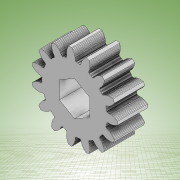
# Autodesk Inventor part: Piñon
Saved by Autodesk Inventor 2022 (Build 260153000, 153)
## iProperties
Created: 2022-03-01
Part Number: Piñon
Material: Genérico
Document SubType Name: Modeling
Designer: Marco
Density: 1 g/cm^3
Appearance: Valor por defecto
Author: Marco
Autodesk Inventor part; units mm, degrees
(part 1 of 2)
ref_plane "YZ Plane" through (0, 0, 0) normal (1, 0, 0) x (0, 1, 0)
ref_plane "XZ Plane" through (0, 0, 0) normal (0, 1, 0) x (-1, 0, 0)
ref_plane "XY Plane" through (0, 0, 0) normal (0, 0, 1) x (1, 0, 0)
sketch "Boceto1" plane through (0, 0, 0) normal (0, 0, 1) x (1, 0, 0)
  line L0 (7.7981, 3.0207) -> (7.6871, 2.8757)
  line L1 (7.6871, 2.8757) -> (7.5784, 2.7454)
  line L2 (7.5784, 2.7454) -> (7.4724, 2.6287)
  line L3 (7.4724, 2.6287) -> (7.3713, 2.5262)
  line L4 (7.3713, 2.5262) -> (7.2722, 2.434)
  line L5 (7.2722, 2.434) -> (7.181, 2.3559)
  line L6 (7.181, 2.3559) -> (7.096, 2.2892)
  line L7 (7.096, 2.2892) -> (7.0182, 2.2331)
  line L8 (7.0182, 2.2331) -> (6.9491, 2.1876)
  line L9 (6.9491, 2.1876) -> (6.8365, 2.1229)
  line L10 (6.8365, 2.1229) -> (6.7437, 2.0808)
  line L11 (6.7437, 2.0808) -> (6.6884, 2.066)
  line L12 (6.6884, 2.066) -> (6.5779, 2.0306)
  line L13 (6.5779, 2.0306) -> (6.4822, 1.9901)
  line L14 (6.4822, 1.9901) -> (6.4013, 1.9458)
  line L15 (6.4013, 1.9458) -> (6.3356, 1.8987)
  line L16 (6.3356, 1.8987) -> (6.285, 1.8501)
  line L17 (6.285, 1.8501) -> (6.2496, 1.8011)
  line L18 (6.2496, 1.8011) -> (6.2375, 1.7768)
  line L19 (6.2375, 1.7768) -> (6.2291, 1.7529)
  line L20 (6.2291, 1.7529) -> (6.2245, 1.7295)
  line L21 (6.2245, 1.7295) -> (6.2236, 1.7067)
  line L22 (6.2236, 1.7067) -> (6.2276, 1.6794)
  line L23 (6.2276, 1.6794) -> (6.2912, 1.423)
  line L24 (6.2912, 1.423) -> (6.3092, 1.3409)
  line L25 (6.3092, 1.3409) -> (6.3262, 1.2585)
  line L26 (6.3262, 1.2585) -> (6.3724, 0.9985)
  line L27 (6.3724, 0.9985) -> (6.3799, 0.9719)
  line L28 (6.3799, 0.9719) -> (6.39, 0.9515)
  line L29 (6.39, 0.9515) -> (6.4037, 0.932)
  line L30 (6.4037, 0.932) -> (6.421, 0.9135)
  line L31 (6.421, 0.9135) -> (6.4419, 0.8963)
  line L32 (6.4419, 0.8963) -> (6.4943, 0.8659)
  line L33 (6.4943, 0.8659) -> (6.5603, 0.8421)
  line L34 (6.5603, 0.8421) -> (6.6395, 0.8258)
  line L35 (6.6395, 0.8258) -> (6.7313, 0.8182)
  line L36 (6.7313, 0.8182) -> (6.8353, 0.8202)
  line L37 (6.8353, 0.8202) -> (6.9506, 0.8328)
  line L38 (6.9506, 0.8328) -> (7.0072, 0.8418)
  line L39 (7.0072, 0.8418) -> (7.1091, 0.8411)
  line L40 (7.1091, 0.8411) -> (7.2382, 0.8277)
  line L41 (7.2382, 0.8277) -> (7.3199, 0.8143)
  line L42 (7.3199, 0.8143) -> (7.4138, 0.7947)
  line L43 (7.4138, 0.7947) -> (7.5185, 0.7683)
  line L44 (7.5185, 0.7683) -> (7.6336, 0.7341)
  line L45 (7.6336, 0.7341) -> (7.7617, 0.6901)
  line L46 (7.7617, 0.6901) -> (7.8957, 0.6377)
  line L47 (7.8957, 0.6377) -> (8.04, 0.5742)
  line L48 (8.04, 0.5742) -> (8.1924, 0.4994)
  line L49 (8.1924, 0.4994) -> (8.3528, 0.4121)
  line L50 (8.3528, 0.4121) -> (8.4937, 0.328)
  arc A0 (8.4937, -0.328) -> (8.4937, 0.328) centre (0, 0) ccw
  line L51 (8.4937, -0.328) -> (8.3525, -0.4122)
  line L52 (8.3525, -0.4122) -> (8.1921, -0.4995)
  line L53 (8.1921, -0.4995) -> (8.0398, -0.5743)
  line L54 (8.0398, -0.5743) -> (7.8955, -0.6378)
  line L55 (7.8955, -0.6378) -> (7.7614, -0.6903)
  line L56 (7.7614, -0.6903) -> (7.6334, -0.7343)
  line L57 (7.6334, -0.7343) -> (7.5183, -0.7685)
  line L58 (7.5183, -0.7685) -> (7.4135, -0.7949)
  line L59 (7.4135, -0.7949) -> (7.3197, -0.8145)
  line L60 (7.3197, -0.8145) -> (7.238, -0.828)
  line L61 (7.238, -0.828) -> (7.1089, -0.8413)
  line L62 (7.1089, -0.8413) -> (7.007, -0.842)
  line L63 (7.007, -0.842) -> (6.9504, -0.8331)
  line L64 (6.9504, -0.8331) -> (6.835, -0.8204)
  line L65 (6.835, -0.8204) -> (6.7311, -0.8184)
  line L66 (6.7311, -0.8184) -> (6.6393, -0.8261)
  line L67 (6.6393, -0.8261) -> (6.5601, -0.8424)
  line L68 (6.5601, -0.8424) -> (6.4941, -0.8662)
  line L69 (6.4941, -0.8662) -> (6.4418, -0.8965)
  line L70 (6.4418, -0.8965) -> (6.4209, -0.9138)
  line L71 (6.4209, -0.9138) -> (6.4035, -0.9322)
  line L72 (6.4035, -0.9322) -> (6.3898, -0.9517)
  line L73 (6.3898, -0.9517) -> (6.3797, -0.9722)
  line L74 (6.3797, -0.9722) -> (6.3722, -0.9988)
  line L75 (6.3722, -0.9988) -> (6.326, -1.2588)
  line L76 (6.326, -1.2588) -> (6.309, -1.3412)
  line L77 (6.309, -1.3412) -> (6.291, -1.4233)
  line L78 (6.291, -1.4233) -> (6.2274, -1.6797)
  line L79 (6.2274, -1.6797) -> (6.2234, -1.707)
  line L80 (6.2234, -1.707) -> (6.2243, -1.7298)
  line L81 (6.2243, -1.7298) -> (6.2289, -1.7532)
  line L82 (6.2289, -1.7532) -> (6.2373, -1.7771)
  line L83 (6.2373, -1.7771) -> (6.2493, -1.8014)
  line L84 (6.2493, -1.8014) -> (6.2848, -1.8503)
  line L85 (6.2848, -1.8503) -> (6.3354, -1.899)
  line L86 (6.3354, -1.899) -> (6.4012, -1.946)
  line L87 (6.4012, -1.946) -> (6.482, -1.9904)
  line L88 (6.482, -1.9904) -> (6.5777, -2.0308)
  line L89 (6.5777, -2.0308) -> (6.6882, -2.0662)
  line L90 (6.6882, -2.0662) -> (6.7436, -2.081)
  line L91 (6.7436, -2.081) -> (6.8364, -2.1231)
  line L92 (6.8364, -2.1231) -> (6.9489, -2.1878)
  line L93 (6.9489, -2.1878) -> (7.0181, -2.2333)
  line L94 (7.0181, -2.2333) -> (7.0959, -2.2894)
  line L95 (7.0959, -2.2894) -> (7.1808, -2.3561)
  line L96 (7.1808, -2.3561) -> (7.2721, -2.4341)
  line L97 (7.2721, -2.4341) -> (7.3712, -2.5264)
  line L98 (7.3712, -2.5264) -> (7.4724, -2.6288)
  line L99 (7.4724, -2.6288) -> (7.5784, -2.7455)
  line L100 (7.5784, -2.7455) -> (7.6871, -2.8758)
  line L101 (7.6871, -2.8758) -> (7.7981, -3.0208)
  line L102 (7.7981, -3.0208) -> (7.8928, -3.155)
  arc A1 (7.626, -3.7543) -> (7.8928, -3.155) centre (0, 0) ccw
  line L103 (7.626, -3.7543) -> (7.4628, -3.7736)
  line L104 (7.4628, -3.7736) -> (7.2808, -3.7881)
  line L105 (7.2808, -3.7881) -> (7.1112, -3.7945)
  line L106 (7.1112, -3.7945) -> (6.9535, -3.7939)
  line L107 (6.9535, -3.7939) -> (6.8097, -3.7873)
  line L108 (6.8097, -3.7873) -> (6.6748, -3.7754)
  line L109 (6.6748, -3.7754) -> (6.5557, -3.7598)
  line L110 (6.5557, -3.7598) -> (6.4493, -3.7414)
  line L111 (6.4493, -3.7414) -> (6.3556, -3.721)
  line L112 (6.3556, -3.721) -> (6.2755, -3.7001)
  line L113 (6.2755, -3.7001) -> (6.1521, -3.6598)
  line L114 (6.1521, -3.6598) -> (6.0587, -3.619)
  line L115 (6.0587, -3.619) -> (6.0106, -3.5878)
  line L116 (6.0106, -3.5878) -> (5.9104, -3.5294)
  line L117 (5.9104, -3.5294) -> (5.8163, -3.4853)
  line L118 (5.8163, -3.4853) -> (5.7293, -3.455)
  line L119 (5.7293, -3.455) -> (5.6503, -3.4376)
  line L120 (5.6503, -3.4376) -> (5.5803, -3.4326)
  line L121 (5.5803, -3.4326) -> (5.5202, -3.439)
  line L122 (5.5202, -3.439) -> (5.4941, -3.4462)
  line L123 (5.4941, -3.4462) -> (5.4707, -3.456)
  line L124 (5.4707, -3.456) -> (5.4502, -3.4683)
  line L125 (5.4502, -3.4683) -> (5.4327, -3.4828)
  line L126 (5.4327, -3.4828) -> (5.4151, -3.5041)
  line L127 (5.4151, -3.5041) -> (5.2671, -3.7229)
  line L128 (5.2671, -3.7229) -> (5.2181, -3.7912)
  line L129 (5.2181, -3.7912) -> (5.1682, -3.8589)
  line L130 (5.1682, -3.8589) -> (5.0059, -4.0673)
  line L131 (5.0059, -4.0673) -> (4.9911, -4.0907)
  line L132 (4.9911, -4.0907) -> (4.9827, -4.1119)
  line L133 (4.9827, -4.1119) -> (4.9774, -4.1351)
  line L134 (4.9774, -4.1351) -> (4.9753, -4.1603)
  line L135 (4.9753, -4.1603) -> (4.9765, -4.1874)
  line L136 (4.9765, -4.1874) -> (4.989, -4.2466)
  line L137 (4.989, -4.2466) -> (5.0154, -4.3116)
  line L138 (5.0154, -4.3116) -> (5.0563, -4.3813)
  line L139 (5.0563, -4.3813) -> (5.1121, -4.4547)
  line L140 (5.1121, -4.4547) -> (5.1831, -4.5306)
  line L141 (5.1831, -4.5306) -> (5.2697, -4.6079)
  line L142 (5.2697, -4.6079) -> (5.3142, -4.6439)
  line L143 (5.3142, -4.6439) -> (5.3819, -4.7201)
  line L144 (5.3819, -4.7201) -> (5.4584, -4.825)
  line L145 (5.4584, -4.825) -> (5.503, -4.8947)
  line L146 (5.503, -4.8947) -> (5.5513, -4.9776)
  line L147 (5.5513, -4.9776) -> (5.6018, -5.0731)
  line L148 (5.6018, -5.0731) -> (5.6534, -5.1815)
  line L149 (5.6534, -5.1815) -> (5.7064, -5.3061)
  line L150 (5.7064, -5.3061) -> (5.7571, -5.4408)
  line L151 (5.7571, -5.4408) -> (5.8065, -5.5905)
  line L152 (5.8065, -5.5905) -> (5.8528, -5.7538)
  line L153 (5.8528, -5.7538) -> (5.8953, -5.9314)
  line L154 (5.8953, -5.9314) -> (5.9271, -6.0925)
  arc A2 (5.4396, -6.5315) -> (5.9271, -6.0925) centre (0, 0) ccw
  line L155 (5.4396, -6.5315) -> (5.2825, -6.4827)
  line L156 (5.2825, -6.4827) -> (5.1103, -6.422)
  line L157 (5.1103, -6.422) -> (4.9528, -6.3588)
  line L158 (4.9528, -6.3588) -> (4.809, -6.2941)
  line L159 (4.809, -6.2941) -> (4.6803, -6.2296)
  line L160 (4.6803, -6.2296) -> (4.562, -6.1639)
  line L161 (4.562, -6.1639) -> (4.4595, -6.1012)
  line L162 (4.4595, -6.1012) -> (4.3698, -6.041)
  line L163 (4.3698, -6.041) -> (4.2925, -5.9843)
  line L164 (4.2925, -5.9843) -> (4.2278, -5.9326)
  line L165 (4.2278, -5.9326) -> (4.1315, -5.8456)
  line L166 (4.1315, -5.8456) -> (4.0628, -5.7704)
  line L167 (4.0628, -5.7704) -> (4.0316, -5.7223)
  line L168 (4.0316, -5.7223) -> (3.9638, -5.6282)
  line L169 (3.9638, -5.6282) -> (3.8957, -5.5496)
  line L170 (3.8957, -5.5496) -> (3.8286, -5.4865)
  line L171 (3.8286, -5.4865) -> (3.7635, -5.4385)
  line L172 (3.7635, -5.4385) -> (3.7016, -5.4054)
  line L173 (3.7016, -5.4054) -> (3.644, -5.3869)
  line L174 (3.644, -5.3869) -> (3.6172, -5.3829)
  line L175 (3.6172, -5.3829) -> (3.5919, -5.3823)
  line L176 (3.5919, -5.3823) -> (3.5682, -5.3852)
  line L177 (3.5682, -5.3852) -> (3.5463, -5.3913)
  line L178 (3.5463, -5.3913) -> (3.5215, -5.4036)
  line L179 (3.5215, -5.4036) -> (3.2974, -5.5433)
  line L180 (3.2974, -5.5433) -> (3.2248, -5.5858)
  line L181 (3.2248, -5.5858) -> (3.1517, -5.6274)
  line L182 (3.1517, -5.6274) -> (2.9187, -5.7518)
  line L183 (2.9187, -5.7518) -> (2.8957, -5.7671)
  line L184 (2.8957, -5.7671) -> (2.8794, -5.783)
  line L185 (2.8794, -5.783) -> (2.8651, -5.8021)
  line L186 (2.8651, -5.8021) -> (2.8529, -5.8243)
  line L187 (2.8529, -5.8243) -> (2.843, -5.8495)
  line L188 (2.843, -5.8495) -> (2.8303, -5.9087)
  line L189 (2.8303, -5.9087) -> (2.8281, -5.9788)
  line L190 (2.8281, -5.9788) -> (2.8371, -6.0592)
  line L191 (2.8371, -6.0592) -> (2.8582, -6.1489)
  line L192 (2.8582, -6.1489) -> (2.8922, -6.2471)
  line L193 (2.8922, -6.2471) -> (2.9398, -6.3529)
  line L194 (2.9398, -6.3529) -> (2.9659, -6.4039)
  line L195 (2.9659, -6.4039) -> (2.9967, -6.501)
  line L196 (2.9967, -6.501) -> (3.0239, -6.628)
  line L197 (3.0239, -6.628) -> (3.0364, -6.7098)
  line L198 (3.0364, -6.7098) -> (3.0468, -6.8051)
  line L199 (3.0468, -6.8051) -> (3.0541, -6.9129)
  line L200 (3.0541, -6.9129) -> (3.0571, -7.033)
  line L201 (3.0571, -7.033) -> (3.0548, -7.1683)
  line L202 (3.0548, -7.1683) -> (3.0464, -7.3121)
  line L203 (3.0464, -7.3121) -> (3.0306, -7.4689)
  line L204 (3.0306, -7.4689) -> (3.0065, -7.6369)
  line L205 (3.0065, -7.6369) -> (2.9731, -7.8164)
  line L206 (2.9731, -7.8164) -> (2.9366, -7.9766)
  arc A3 (2.3128, -8.1793) -> (2.9366, -7.9766) centre (0, 0) ccw
  line L207 (2.3128, -8.1793) -> (2.1908, -8.0711)
  line L208 (2.1908, -8.0711) -> (2.0582, -7.9456)
  line L209 (2.0582, -7.9456) -> (1.94, -7.8238)
  line L210 (1.94, -7.8238) -> (1.835, -7.7062)
  line L211 (1.835, -7.7062) -> (1.7437, -7.5949)
  line L212 (1.7437, -7.5949) -> (1.6623, -7.4867)
  line L213 (1.6623, -7.4867) -> (1.5942, -7.3878)
  line L214 (1.5942, -7.3878) -> (1.5367, -7.2963)
  line L215 (1.5367, -7.2963) -> (1.4891, -7.2131)
  line L216 (1.4891, -7.2131) -> (1.4511, -7.1396)
  line L217 (1.4511, -7.1396) -> (1.3985, -7.0209)
  line L218 (1.3985, -7.0209) -> (1.3663, -6.9242)
  line L219 (1.3663, -6.9242) -> (1.3573, -6.8676)
  line L220 (1.3573, -6.8676) -> (1.3337, -6.754)
  line L221 (1.3337, -6.754) -> (1.3034, -6.6546)
  line L222 (1.3034, -6.6546) -> (1.2678, -6.5696)
  line L223 (1.2678, -6.5696) -> (1.2278, -6.4993)
  line L224 (1.2278, -6.4993) -> (1.1847, -6.4439)
  line L225 (1.1847, -6.4439) -> (1.1397, -6.4035)
  line L226 (1.1397, -6.4035) -> (1.1169, -6.389)
  line L227 (1.1169, -6.389) -> (1.094, -6.3782)
  line L228 (1.094, -6.3782) -> (1.0712, -6.3711)
  line L229 (1.0712, -6.3711) -> (1.0486, -6.3678)
  line L230 (1.0486, -6.3678) -> (1.021, -6.369)
  line L231 (1.021, -6.369) -> (0.7594, -6.4054)
  line L232 (0.7594, -6.4054) -> (0.6758, -6.4147)
  line L233 (0.6758, -6.4147) -> (0.5922, -6.423)
  line L234 (0.5922, -6.423) -> (0.3287, -6.4418)
  line L235 (0.3287, -6.4418) -> (0.3014, -6.4464)
  line L236 (0.3014, -6.4464) -> (0.2801, -6.4543)
  line L237 (0.2801, -6.4543) -> (0.2592, -6.4659)
  line L238 (0.2592, -6.4659) -> (0.2391, -6.4813)
  line L239 (0.2391, -6.4813) -> (0.2197, -6.5002)
  line L240 (0.2197, -6.5002) -> (0.1841, -6.5491)
  line L241 (0.1841, -6.5491) -> (0.1535, -6.6123)
  line L242 (0.1535, -6.6123) -> (0.1291, -6.6893)
  line L243 (0.1291, -6.6893) -> (0.1119, -6.7799)
  line L244 (0.1119, -6.7799) -> (0.103, -6.8834)
  line L245 (0.103, -6.8834) -> (0.1034, -6.9994)
  line L246 (0.1034, -6.9994) -> (0.1065, -7.0567)
  line L247 (0.1065, -7.0567) -> (0.0951, -7.1579)
  line L248 (0.0951, -7.1579) -> (0.0683, -7.285)
  line L249 (0.0683, -7.285) -> (0.0464, -7.3648)
  line L250 (0.0464, -7.3648) -> (0.0172, -7.4561)
  line L251 (0.0172, -7.4561) -> (-0.02, -7.5575)
  line L252 (-0.02, -7.5575) -> (-0.0661, -7.6685)
  line L253 (-0.0661, -7.6685) -> (-0.1232, -7.7912)
  line L254 (-0.1232, -7.7912) -> (-0.1894, -7.919)
  line L255 (-0.1894, -7.919) -> (-0.2676, -8.0559)
  line L256 (-0.2676, -8.0559) -> (-0.3579, -8.1996)
  line L257 (-0.3579, -8.1996) -> (-0.4615, -8.35)
  line L258 (-0.4615, -8.35) -> (-0.5599, -8.4815)
  arc A4 (-1.2139, -8.4129) -> (-0.5599, -8.4815) centre (0, 0) ccw
  line L259 (-1.2139, -8.4129) -> (-1.283, -8.2636)
  line L260 (-1.283, -8.2636) -> (-1.353, -8.0949)
  line L261 (-1.353, -8.0949) -> (-1.4115, -7.9356)
  line L262 (-1.4115, -7.9356) -> (-1.4595, -7.7855)
  line L263 (-1.4595, -7.7855) -> (-1.4977, -7.6466)
  line L264 (-1.4977, -7.6466) -> (-1.528, -7.5147)
  line L265 (-1.528, -7.5147) -> (-1.55, -7.3966)
  line L266 (-1.55, -7.3966) -> (-1.5653, -7.2897)
  line L267 (-1.5653, -7.2897) -> (-1.5749, -7.1943)
  line L268 (-1.5749, -7.1943) -> (-1.5798, -7.1116)
  line L269 (-1.5798, -7.1116) -> (-1.5796, -6.9818)
  line L270 (-1.5796, -6.9818) -> (-1.5697, -6.8804)
  line L271 (-1.5697, -6.8804) -> (-1.5548, -6.8251)
  line L272 (-1.5548, -6.8251) -> (-1.5302, -6.7117)
  line L273 (-1.5302, -6.7117) -> (-1.5174, -6.6086)
  line L274 (-1.5174, -6.6086) -> (-1.5154, -6.5164)
  line L275 (-1.5154, -6.5164) -> (-1.5234, -6.4359)
  line L276 (-1.5234, -6.4359) -> (-1.5402, -6.3678)
  line L277 (-1.5402, -6.3678) -> (-1.5649, -6.3126)
  line L278 (-1.5649, -6.3126) -> (-1.5798, -6.29)
  line L279 (-1.5798, -6.29) -> (-1.5964, -6.2708)
  line L280 (-1.5964, -6.2708) -> (-1.6143, -6.2551)
  line L281 (-1.6143, -6.2551) -> (-1.6336, -6.2429)
  line L282 (-1.6336, -6.2429) -> (-1.6593, -6.2328)
  line L283 (-1.6593, -6.2328) -> (-1.9131, -6.1596)
  line L284 (-1.9131, -6.1596) -> (-1.9932, -6.1342)
  line L285 (-1.9932, -6.1342) -> (-2.073, -6.1077)
  line L286 (-2.073, -6.1077) -> (-2.3214, -6.0177)
  line L287 (-2.3214, -6.0177) -> (-2.3482, -6.0109)
  line L288 (-2.3482, -6.0109) -> (-2.3709, -6.0094)
  line L289 (-2.3709, -6.0094) -> (-2.3947, -6.0116)
  line L290 (-2.3947, -6.0116) -> (-2.4193, -6.0174)
  line L291 (-2.4193, -6.0174) -> (-2.4447, -6.0269)
  line L292 (-2.4447, -6.0269) -> (-2.4971, -6.057)
  line L293 (-2.4971, -6.057) -> (-2.5507, -6.1023)
  line L294 (-2.5507, -6.1023) -> (-2.6044, -6.1627)
  line L295 (-2.6044, -6.1627) -> (-2.657, -6.2385)
  line L296 (-2.657, -6.2385) -> (-2.7072, -6.3295)
  line L297 (-2.7072, -6.3295) -> (-2.7539, -6.4356)
  line L298 (-2.7539, -6.4356) -> (-2.7745, -6.4891)
  line L299 (-2.7745, -6.4891) -> (-2.826, -6.577)
  line L300 (-2.826, -6.577) -> (-2.9021, -6.6822)
  line L301 (-2.9021, -6.6822) -> (-2.9546, -6.7462)
  line L302 (-2.9546, -6.7462) -> (-3.0185, -6.8178)
  line L303 (-3.0185, -6.8178) -> (-3.0937, -6.8953)
  line L304 (-3.0937, -6.8953) -> (-3.1809, -6.9779)
  line L305 (-3.1809, -6.9779) -> (-3.283, -7.0668)
  line L306 (-3.283, -7.0668) -> (-3.3955, -7.1566)
  line L307 (-3.3955, -7.1566) -> (-3.5226, -7.2499)
  line L308 (-3.5226, -7.2499) -> (-3.6636, -7.3444)
  line L309 (-3.6636, -7.3444) -> (-3.8194, -7.4396)
  line L310 (-3.8194, -7.4396) -> (-3.9628, -7.5197)
  arc A5 (-4.5309, -7.1917) -> (-3.9628, -7.5197) centre (0, 0) ccw
  line L311 (-4.5309, -7.1917) -> (-4.5332, -7.0275)
  line L312 (-4.5332, -7.0275) -> (-4.5286, -6.8449)
  line L313 (-4.5286, -6.8449) -> (-4.5172, -6.6756)
  line L314 (-4.5172, -6.6756) -> (-4.5001, -6.5189)
  line L315 (-4.5001, -6.5189) -> (-4.4785, -6.3766)
  line L316 (-4.4785, -6.3766) -> (-4.4526, -6.2437)
  line L317 (-4.4526, -6.2437) -> (-4.4246, -6.1269)
  line L318 (-4.4246, -6.1269) -> (-4.3951, -6.023)
  line L319 (-4.3951, -6.023) -> (-4.3651, -5.9319)
  line L320 (-4.3651, -5.9319) -> (-4.3359, -5.8544)
  line L321 (-4.3359, -5.8544) -> (-4.2829, -5.7359)
  line L322 (-4.2829, -5.7359) -> (-4.2326, -5.6473)
  line L323 (-4.2326, -5.6473) -> (-4.1965, -5.6028)
  line L324 (-4.1965, -5.6028) -> (-4.1279, -5.5092)
  line L325 (-4.1279, -5.5092) -> (-4.0742, -5.4202)
  line L326 (-4.0742, -5.4202) -> (-4.035, -5.3369)
  line L327 (-4.035, -5.3369) -> (-4.0094, -5.2601)
  line L328 (-4.0094, -5.2601) -> (-3.9971, -5.1911)
  line L329 (-3.9971, -5.1911) -> (-3.9966, -5.1312)
  line L330 (-3.9966, -5.1312) -> (-4.001, -5.1045)
  line L331 (-4.001, -5.1045) -> (-4.0083, -5.0803)
  line L332 (-4.0083, -5.0803) -> (-4.0184, -5.0586)
  line L333 (-4.0184, -5.0586) -> (-4.031, -5.0396)
  line L334 (-4.031, -5.0396) -> (-4.0503, -5.0199)
  line L335 (-4.0503, -5.0199) -> (-4.2524, -4.8498)
  line L336 (-4.2524, -4.8498) -> (-4.3153, -4.794)
  line L337 (-4.3153, -4.794) -> (-4.3774, -4.7373)
  line L338 (-4.3774, -4.7373) -> (-4.5677, -4.5541)
  line L339 (-4.5677, -4.5541) -> (-4.5893, -4.5369)
  line L340 (-4.5893, -4.5369) -> (-4.6095, -4.5264)
  line L341 (-4.6095, -4.5264) -> (-4.6321, -4.5187)
  line L342 (-4.6321, -4.5187) -> (-4.657, -4.5139)
  line L343 (-4.657, -4.5139) -> (-4.684, -4.5123)
  line L344 (-4.684, -4.5123) -> (-4.7442, -4.5185)
  line L345 (-4.7442, -4.5185) -> (-4.8116, -4.538)
  line L346 (-4.8116, -4.538) -> (-4.8852, -4.5714)
  line L347 (-4.8852, -4.5714) -> (-4.964, -4.6192)
  line L348 (-4.964, -4.6192) -> (-5.0469, -4.6819)
  line L349 (-5.0469, -4.6819) -> (-5.1328, -4.7599)
  line L350 (-5.1328, -4.7599) -> (-5.1733, -4.8004)
  line L351 (-5.1733, -4.8004) -> (-5.2562, -4.8597)
  line L352 (-5.2562, -4.8597) -> (-5.3685, -4.9249)
  line L353 (-5.3685, -4.9249) -> (-5.4425, -4.962)
  line L354 (-5.4425, -4.962) -> (-5.5299, -5.0014)
  line L355 (-5.5299, -5.0014) -> (-5.6301, -5.0416)
  line L356 (-5.6301, -5.0416) -> (-5.7434, -5.0816)
  line L357 (-5.7434, -5.0816) -> (-5.8728, -5.1213)
  line L358 (-5.8728, -5.1213) -> (-6.0121, -5.1577)
  line L359 (-6.0121, -5.1577) -> (-6.1662, -5.1911)
  line L360 (-6.1662, -5.1911) -> (-6.3334, -5.2201)
  line L361 (-6.3334, -5.2201) -> (-6.5144, -5.2438)
  line L362 (-6.5144, -5.2438) -> (-6.678, -5.2587)
  arc A6 (-7.0642, -4.7273) -> (-6.678, -5.2587) centre (0, 0) ccw
  line L363 (-7.0642, -4.7273) -> (-6.9995, -4.5763)
  line L364 (-6.9995, -4.5763) -> (-6.9211, -4.4114)
  line L365 (-6.9211, -4.4114) -> (-6.8418, -4.2613)
  line L366 (-6.8418, -4.2613) -> (-6.7625, -4.1251)
  line L367 (-6.7625, -4.1251) -> (-6.6849, -4.0039)
  line L368 (-6.6849, -4.0039) -> (-6.6071, -3.893)
  line L369 (-6.6071, -3.893) -> (-6.5341, -3.7977)
  line L370 (-6.5341, -3.7977) -> (-6.4649, -3.7147)
  line L371 (-6.4649, -3.7147) -> (-6.4005, -3.6437)
  line L372 (-6.4005, -3.6437) -> (-6.3423, -3.5848)
  line L373 (-6.3423, -3.5848) -> (-6.2457, -3.4981)
  line L374 (-6.2457, -3.4981) -> (-6.1637, -3.4376)
  line L375 (-6.1637, -3.4376) -> (-6.1126, -3.4116)
  line L376 (-6.1126, -3.4116) -> (-6.0119, -3.354)
  line L377 (-6.0119, -3.354) -> (-5.9267, -3.2945)
  line L378 (-5.9267, -3.2945) -> (-5.8569, -3.2343)
  line L379 (-5.8569, -3.2343) -> (-5.8024, -3.1746)
  line L380 (-5.8024, -3.1746) -> (-5.763, -3.1165)
  line L381 (-5.763, -3.1165) -> (-5.7385, -3.0612)
  line L382 (-5.7385, -3.0612) -> (-5.7317, -3.035)
  line L383 (-5.7317, -3.035) -> (-5.7285, -3.0099)
  line L384 (-5.7285, -3.0099) -> (-5.7287, -2.9859)
  line L385 (-5.7287, -2.9859) -> (-5.7325, -2.9634)
  line L386 (-5.7325, -2.9634) -> (-5.7421, -2.9375)
  line L387 (-5.7421, -2.9375) -> (-5.8576, -2.7)
  line L388 (-5.8576, -2.7) -> (-5.8923, -2.6234)
  line L389 (-5.8923, -2.6234) -> (-5.9261, -2.5464)
  line L390 (-5.9261, -2.5464) -> (-6.0254, -2.3016)
  line L391 (-6.0254, -2.3016) -> (-6.0382, -2.2771)
  line L392 (-6.0382, -2.2771) -> (-6.0523, -2.2593)
  line L393 (-6.0523, -2.2593) -> (-6.0698, -2.243)
  line L394 (-6.0698, -2.243) -> (-6.0906, -2.2286)
  line L395 (-6.0906, -2.2286) -> (-6.1147, -2.2161)
  line L396 (-6.1147, -2.2161) -> (-6.1721, -2.1973)
  line L397 (-6.1721, -2.1973) -> (-6.2417, -2.1877)
  line L398 (-6.2417, -2.1877) -> (-6.3225, -2.1883)
  line L399 (-6.3225, -2.1883) -> (-6.414, -2.1999)
  line L400 (-6.414, -2.1999) -> (-6.5152, -2.2235)
  line L401 (-6.5152, -2.2235) -> (-6.6254, -2.2598)
  line L402 (-6.6254, -2.2598) -> (-6.6789, -2.2803)
  line L403 (-6.6789, -2.2803) -> (-6.7787, -2.3008)
  line L404 (-6.7787, -2.3008) -> (-6.9078, -2.3146)
  line L405 (-6.9078, -2.3146) -> (-6.9905, -2.3184)
  line L406 (-6.9905, -2.3184) -> (-7.0864, -2.3188)
  line L407 (-7.0864, -2.3188) -> (-7.1943, -2.3148)
  line L408 (-7.1943, -2.3148) -> (-7.314, -2.3053)
  line L409 (-7.314, -2.3053) -> (-7.4484, -2.2889)
  line L410 (-7.4484, -2.2889) -> (-7.5904, -2.2654)
  line L411 (-7.5904, -2.2654) -> (-7.7448, -2.2333)
  line L412 (-7.7448, -2.2333) -> (-7.9093, -2.1918)
  line L413 (-7.9093, -2.1918) -> (-8.0844, -2.1398)
  line L414 (-8.0844, -2.1398) -> (-8.2399, -2.0868)
  arc A7 (-8.3763, -1.4451) -> (-8.2399, -2.0868) centre (0, 0) ccw
  line L415 (-8.3763, -1.4451) -> (-8.2557, -1.3335)
  line L416 (-8.2557, -1.3335) -> (-8.117, -1.2148)
  line L417 (-8.117, -1.2148) -> (-7.9836, -1.1099)
  line L418 (-7.9836, -1.1099) -> (-7.8556, -1.0178)
  line L419 (-7.8556, -1.0178) -> (-7.7354, -0.9386)
  line L420 (-7.7354, -0.9386) -> (-7.6193, -0.8689)
  line L421 (-7.6193, -0.8689) -> (-7.5138, -0.8115)
  line L422 (-7.5138, -0.8115) -> (-7.4169, -0.7639)
  line L423 (-7.4169, -0.7639) -> (-7.3291, -0.7253)
  line L424 (-7.3291, -0.7253) -> (-7.252, -0.6951)
  line L425 (-7.252, -0.6951) -> (-7.1285, -0.6552)
  line L426 (-7.1285, -0.6552) -> (-7.0289, -0.6334)
  line L427 (-7.0289, -0.6334) -> (-6.9717, -0.6304)
  line L428 (-6.9717, -0.6304) -> (-6.8563, -0.6188)
  line L429 (-6.8563, -0.6188) -> (-6.7542, -0.5991)
  line L430 (-6.7542, -0.5991) -> (-6.666, -0.5725)
  line L431 (-6.666, -0.5725) -> (-6.5919, -0.5401)
  line L432 (-6.5919, -0.5401) -> (-6.5323, -0.5031)
  line L433 (-6.5323, -0.5031) -> (-6.4874, -0.4625)
  line L434 (-6.4874, -0.4625) -> (-6.4705, -0.4413)
  line L435 (-6.4705, -0.4413) -> (-6.4574, -0.4197)
  line L436 (-6.4574, -0.4197) -> (-6.448, -0.3977)
  line L437 (-6.448, -0.3977) -> (-6.4424, -0.3757)
  line L438 (-6.4424, -0.3757) -> (-6.4406, -0.3481)
  line L439 (-6.4406, -0.3481) -> (-6.4495, -0.0841)
  line L440 (-6.4495, -0.0841) -> (-6.45, 0)
  line L441 (-6.45, 0) -> (-6.4495, 0.0841)
  line L442 (-6.4495, 0.0841) -> (-6.4406, 0.3481)
  line L443 (-6.4406, 0.3481) -> (-6.4423, 0.3756)
  line L444 (-6.4423, 0.3756) -> (-6.448, 0.3977)
  line L445 (-6.448, 0.3977) -> (-6.4574, 0.4196)
  line L446 (-6.4574, 0.4196) -> (-6.4705, 0.4413)
  line L447 (-6.4705, 0.4413) -> (-6.4873, 0.4625)
  line L448 (-6.4873, 0.4625) -> (-6.5322, 0.503)
  line L449 (-6.5322, 0.503) -> (-6.5918, 0.5401)
  line L450 (-6.5918, 0.5401) -> (-6.6659, 0.5725)
  line L451 (-6.6659, 0.5725) -> (-6.7542, 0.5991)
  line L452 (-6.7542, 0.5991) -> (-6.8562, 0.6187)
  line L453 (-6.8562, 0.6187) -> (-6.9716, 0.6303)
  line L454 (-6.9716, 0.6303) -> (-7.0289, 0.6333)
  line L455 (-7.0289, 0.6333) -> (-7.1284, 0.6552)
  line L456 (-7.1284, 0.6552) -> (-7.2519, 0.6951)
  line L457 (-7.2519, 0.6951) -> (-7.3291, 0.7253)
  line L458 (-7.3291, 0.7253) -> (-7.4168, 0.7639)
  line L459 (-7.4168, 0.7639) -> (-7.5138, 0.8115)
  line L460 (-7.5138, 0.8115) -> (-7.6193, 0.8689)
  line L461 (-7.6193, 0.8689) -> (-7.7354, 0.9385)
  line L462 (-7.7354, 0.9385) -> (-7.8556, 1.0177)
  line L463 (-7.8556, 1.0177) -> (-7.9836, 1.1098)
  line L464 (-7.9836, 1.1098) -> (-8.117, 1.2146)
  line L465 (-8.117, 1.2146) -> (-8.2558, 1.3333)
  line L466 (-8.2558, 1.3333) -> (-8.3763, 1.445)
  arc A8 (-8.2401, 2.0859) -> (-8.3763, 1.445) centre (0, 0) ccw
  line L467 (-8.2401, 2.0859) -> (-8.0846, 2.1389)
  line L468 (-8.0846, 2.1389) -> (-7.9096, 2.1909)
  line L469 (-7.9096, 2.1909) -> (-7.745, 2.2324)
  line L470 (-7.745, 2.2324) -> (-7.5907, 2.2646)
  line L471 (-7.5907, 2.2646) -> (-7.4486, 2.288)
  line L472 (-7.4486, 2.288) -> (-7.3143, 2.3045)
  line L473 (-7.3143, 2.3045) -> (-7.1945, 2.314)
  line L474 (-7.1945, 2.314) -> (-7.0866, 2.3181)
  line L475 (-7.0866, 2.3181) -> (-6.9907, 2.3177)
  line L476 (-6.9907, 2.3177) -> (-6.908, 2.3139)
  line L477 (-6.908, 2.3139) -> (-6.7789, 2.3001)
  line L478 (-6.7789, 2.3001) -> (-6.6791, 2.2796)
  line L479 (-6.6791, 2.2796) -> (-6.6256, 2.2591)
  line L480 (-6.6256, 2.2591) -> (-6.5154, 2.2228)
  line L481 (-6.5154, 2.2228) -> (-6.4142, 2.1992)
  line L482 (-6.4142, 2.1992) -> (-6.3228, 2.1876)
  line L483 (-6.3228, 2.1876) -> (-6.2419, 2.1871)
  line L484 (-6.2419, 2.1871) -> (-6.1724, 2.1967)
  line L485 (-6.1724, 2.1967) -> (-6.1149, 2.2155)
  line L486 (-6.1149, 2.2155) -> (-6.0909, 2.228)
  line L487 (-6.0909, 2.228) -> (-6.0701, 2.2424)
  line L488 (-6.0701, 2.2424) -> (-6.0526, 2.2587)
  line L489 (-6.0526, 2.2587) -> (-6.0385, 2.2765)
  line L490 (-6.0385, 2.2765) -> (-6.0256, 2.301)
  line L491 (-6.0256, 2.301) -> (-5.9264, 2.5458)
  line L492 (-5.9264, 2.5458) -> (-5.8927, 2.6228)
  line L493 (-5.8927, 2.6228) -> (-5.858, 2.6994)
  line L494 (-5.858, 2.6994) -> (-5.7425, 2.937)
  line L495 (-5.7425, 2.937) -> (-5.7329, 2.9629)
  line L496 (-5.7329, 2.9629) -> (-5.7291, 2.9854)
  line L497 (-5.7291, 2.9854) -> (-5.7288, 3.0092)
  line L498 (-5.7288, 3.0092) -> (-5.732, 3.0343)
  line L499 (-5.732, 3.0343) -> (-5.7388, 3.0606)
  line L500 (-5.7388, 3.0606) -> (-5.7633, 3.1158)
  line L501 (-5.7633, 3.1158) -> (-5.8027, 3.1739)
  line L502 (-5.8027, 3.1739) -> (-5.8572, 3.2336)
  line L503 (-5.8572, 3.2336) -> (-5.927, 3.2938)
  line L504 (-5.927, 3.2938) -> (-6.0122, 3.3533)
  line L505 (-6.0122, 3.3533) -> (-6.113, 3.4108)
  line L506 (-6.113, 3.4108) -> (-6.164, 3.4368)
  line L507 (-6.164, 3.4368) -> (-6.2461, 3.4973)
  line L508 (-6.2461, 3.4973) -> (-6.3427, 3.584)
  line L509 (-6.3427, 3.584) -> (-6.4009, 3.6429)
  line L510 (-6.4009, 3.6429) -> (-6.4653, 3.7139)
  line L511 (-6.4653, 3.7139) -> (-6.5346, 3.7968)
  line L512 (-6.5346, 3.7968) -> (-6.6076, 3.8921)
  line L513 (-6.6076, 3.8921) -> (-6.6853, 4.003)
  line L514 (-6.6853, 4.003) -> (-6.763, 4.1242)
  line L515 (-6.763, 4.1242) -> (-6.8424, 4.2604)
  line L516 (-6.8424, 4.2604) -> (-6.9217, 4.4104)
  line L517 (-6.9217, 4.4104) -> (-7.0001, 4.5753)
  line L518 (-7.0001, 4.5753) -> (-7.0648, 4.7263)
  arc A9 (-6.6793, 5.2571) -> (-7.0648, 4.7263) centre (0, 0) ccw
  line L519 (-6.6793, 5.2571) -> (-6.5157, 5.2423)
  line L520 (-6.5157, 5.2423) -> (-6.3346, 5.2186)
  line L521 (-6.3346, 5.2186) -> (-6.1674, 5.1896)
  line L522 (-6.1674, 5.1896) -> (-6.0133, 5.1562)
  line L523 (-6.0133, 5.1562) -> (-5.874, 5.1199)
  line L524 (-5.874, 5.1199) -> (-5.7446, 5.0802)
  line L525 (-5.7446, 5.0802) -> (-5.6313, 5.0402)
  line L526 (-5.6313, 5.0402) -> (-5.5311, 5)
  line L527 (-5.5311, 5) -> (-5.4437, 4.9607)
  line L528 (-5.4437, 4.9607) -> (-5.3696, 4.9236)
  line L529 (-5.3696, 4.9236) -> (-5.2573, 4.8585)
  line L530 (-5.2573, 4.8585) -> (-5.1745, 4.7992)
  line L531 (-5.1745, 4.7992) -> (-5.1339, 4.7586)
  line L532 (-5.1339, 4.7586) -> (-5.0481, 4.6807)
  line L533 (-5.0481, 4.6807) -> (-4.9651, 4.618)
  line L534 (-4.9651, 4.618) -> (-4.8863, 4.5702)
  line L535 (-4.8863, 4.5702) -> (-4.8127, 4.5368)
  line L536 (-4.8127, 4.5368) -> (-4.7453, 4.5173)
  line L537 (-4.7453, 4.5173) -> (-4.6851, 4.5111)
  line L538 (-4.6851, 4.5111) -> (-4.6581, 4.5127)
  line L539 (-4.6581, 4.5127) -> (-4.6332, 4.5175)
  line L540 (-4.6332, 4.5175) -> (-4.6106, 4.5252)
  line L541 (-4.6106, 4.5252) -> (-4.5904, 4.5357)
  line L542 (-4.5904, 4.5357) -> (-4.5688, 4.5529)
  line L543 (-4.5688, 4.5529) -> (-4.3785, 4.7361)
  line L544 (-4.3785, 4.7361) -> (-4.3164, 4.7928)
  line L545 (-4.3164, 4.7928) -> (-4.2535, 4.8486)
  line L546 (-4.2535, 4.8486) -> (-4.0514, 5.0187)
  line L547 (-4.0514, 5.0187) -> (-4.0321, 5.0385)
  line L548 (-4.0321, 5.0385) -> (-4.0195, 5.0574)
  line L549 (-4.0195, 5.0574) -> (-4.0095, 5.0791)
  line L550 (-4.0095, 5.0791) -> (-4.0021, 5.1033)
  line L551 (-4.0021, 5.1033) -> (-3.9977, 5.13)
  line L552 (-3.9977, 5.13) -> (-3.9977, 5.1906)
  line L553 (-3.9977, 5.1906) -> (-4.01, 5.2597)
  line L554 (-4.01, 5.2597) -> (-4.0355, 5.3364)
  line L555 (-4.0355, 5.3364) -> (-4.0748, 5.4198)
  line L556 (-4.0748, 5.4198) -> (-4.1285, 5.5088)
  line L557 (-4.1285, 5.5088) -> (-4.1971, 5.6024)
  line L558 (-4.1971, 5.6024) -> (-4.2331, 5.6469)
  line L559 (-4.2331, 5.6469) -> (-4.2835, 5.7355)
  line L560 (-4.2835, 5.7355) -> (-4.3365, 5.854)
  line L561 (-4.3365, 5.854) -> (-4.3657, 5.9315)
  line L562 (-4.3657, 5.9315) -> (-4.3957, 6.0226)
  line L563 (-4.3957, 6.0226) -> (-4.4252, 6.1265)
  line L564 (-4.4252, 6.1265) -> (-4.4532, 6.2433)
  line L565 (-4.4532, 6.2433) -> (-4.4791, 6.3761)
  line L566 (-4.4791, 6.3761) -> (-4.5007, 6.5185)
  line L567 (-4.5007, 6.5185) -> (-4.5179, 6.6752)
  line L568 (-4.5179, 6.6752) -> (-4.5292, 6.8445)
  line L569 (-4.5292, 6.8445) -> (-4.5339, 7.0271)
  line L570 (-4.5339, 7.0271) -> (-4.5316, 7.1913)
  arc A10 (-3.9636, 7.5193) -> (-4.5316, 7.1913) centre (0, 0) ccw
  line L571 (-3.9636, 7.5193) -> (-3.8201, 7.4392)
  line L572 (-3.8201, 7.4392) -> (-3.6644, 7.344)
  line L573 (-3.6644, 7.344) -> (-3.5234, 7.2495)
  line L574 (-3.5234, 7.2495) -> (-3.3963, 7.1563)
  line L575 (-3.3963, 7.1563) -> (-3.2838, 7.0664)
  line L576 (-3.2838, 7.0664) -> (-3.1817, 6.9775)
  line L577 (-3.1817, 6.9775) -> (-3.0945, 6.8949)
  line L578 (-3.0945, 6.8949) -> (-3.0193, 6.8174)
  line L579 (-3.0193, 6.8174) -> (-2.9554, 6.7458)
  line L580 (-2.9554, 6.7458) -> (-2.9029, 6.6818)
  line L581 (-2.9029, 6.6818) -> (-2.8268, 6.5767)
  line L582 (-2.8268, 6.5767) -> (-2.7753, 6.4887)
  line L583 (-2.7753, 6.4887) -> (-2.7547, 6.4352)
  line L584 (-2.7547, 6.4352) -> (-2.708, 6.3291)
  line L585 (-2.708, 6.3291) -> (-2.6578, 6.2381)
  line L586 (-2.6578, 6.2381) -> (-2.6052, 6.1624)
  line L587 (-2.6052, 6.1624) -> (-2.5515, 6.1019)
  line L588 (-2.5515, 6.1019) -> (-2.4978, 6.0567)
  line L589 (-2.4978, 6.0567) -> (-2.4454, 6.0265)
  line L590 (-2.4454, 6.0265) -> (-2.42, 6.0171)
  line L591 (-2.42, 6.0171) -> (-2.3954, 6.0113)
  line L592 (-2.3954, 6.0113) -> (-2.3716, 6.0091)
  line L593 (-2.3716, 6.0091) -> (-2.3489, 6.0106)
  line L594 (-2.3489, 6.0106) -> (-2.3221, 6.0174)
  line L595 (-2.3221, 6.0174) -> (-2.0738, 6.1075)
  line L596 (-2.0738, 6.1075) -> (-1.994, 6.134)
  line L597 (-1.994, 6.134) -> (-1.9139, 6.1594)
  line L598 (-1.9139, 6.1594) -> (-1.6601, 6.2326)
  line L599 (-1.6601, 6.2326) -> (-1.6344, 6.2428)
  line L600 (-1.6344, 6.2428) -> (-1.6151, 6.255)
  line L601 (-1.6151, 6.255) -> (-1.5972, 6.2707)
  line L602 (-1.5972, 6.2707) -> (-1.5806, 6.2899)
  line L603 (-1.5806, 6.2899) -> (-1.5657, 6.3125)
  line L604 (-1.5657, 6.3125) -> (-1.541, 6.3677)
  line L605 (-1.541, 6.3677) -> (-1.5242, 6.4358)
  line L606 (-1.5242, 6.4358) -> (-1.5163, 6.5163)
  line L607 (-1.5163, 6.5163) -> (-1.5183, 6.6084)
  line L608 (-1.5183, 6.6084) -> (-1.5311, 6.7116)
  line L609 (-1.5311, 6.7116) -> (-1.5557, 6.8249)
  line L610 (-1.5557, 6.8249) -> (-1.5706, 6.8803)
  line L611 (-1.5706, 6.8803) -> (-1.5805, 6.9817)
  line L612 (-1.5805, 6.9817) -> (-1.5808, 7.1115)
  line L613 (-1.5808, 7.1115) -> (-1.5759, 7.1942)
  line L614 (-1.5759, 7.1942) -> (-1.5663, 7.2896)
  line L615 (-1.5663, 7.2896) -> (-1.551, 7.3965)
  line L616 (-1.551, 7.3965) -> (-1.529, 7.5146)
  line L617 (-1.529, 7.5146) -> (-1.4987, 7.6465)
  line L618 (-1.4987, 7.6465) -> (-1.4605, 7.7853)
  line L619 (-1.4605, 7.7853) -> (-1.4125, 7.9355)
  line L620 (-1.4125, 7.9355) -> (-1.354, 8.0948)
  line L621 (-1.354, 8.0948) -> (-1.284, 8.2634)
  line L622 (-1.284, 8.2634) -> (-1.2149, 8.4127)
  arc A11 (-0.5625, 8.4814) -> (-1.2149, 8.4127) centre (0, 0) ccw
  line L623 (-0.5625, 8.4814) -> (-0.4641, 8.3499)
  line L624 (-0.4641, 8.3499) -> (-0.3605, 8.1995)
  line L625 (-0.3605, 8.1995) -> (-0.2702, 8.0558)
  line L626 (-0.2702, 8.0558) -> (-0.1919, 7.919)
  line L627 (-0.1919, 7.919) -> (-0.1257, 7.7911)
  line L628 (-0.1257, 7.7911) -> (-0.0686, 7.6684)
  line L629 (-0.0686, 7.6684) -> (-0.0225, 7.5575)
  line L630 (-0.0225, 7.5575) -> (0.0147, 7.4561)
  line L631 (0.0147, 7.4561) -> (0.0439, 7.3648)
  line L632 (0.0439, 7.3648) -> (0.0659, 7.2849)
  line L633 (0.0659, 7.2849) -> (0.0926, 7.1579)
  line L634 (0.0926, 7.1579) -> (0.104, 7.0566)
  line L635 (0.104, 7.0566) -> (0.101, 6.9994)
  line L636 (0.101, 6.9994) -> (0.1005, 6.8834)
  line L637 (0.1005, 6.8834) -> (0.1094, 6.7798)
  line L638 (0.1094, 6.7798) -> (0.1266, 6.6893)
  line L639 (0.1266, 6.6893) -> (0.1511, 6.6122)
  line L640 (0.1511, 6.6122) -> (0.1817, 6.5491)
  line L641 (0.1817, 6.5491) -> (0.2173, 6.5002)
  line L642 (0.2173, 6.5002) -> (0.2366, 6.4812)
  line L643 (0.2366, 6.4812) -> (0.2568, 6.4659)
  line L644 (0.2568, 6.4659) -> (0.2776, 6.4543)
  line L645 (0.2776, 6.4543) -> (0.299, 6.4463)
  line L646 (0.299, 6.4463) -> (0.3262, 6.4417)
  line L647 (0.3262, 6.4417) -> (0.5897, 6.4229)
  line L648 (0.5897, 6.4229) -> (0.6734, 6.4146)
  line L649 (0.6734, 6.4146) -> (0.7569, 6.4053)
  line L650 (0.7569, 6.4053) -> (1.0186, 6.3689)
  line L651 (1.0186, 6.3689) -> (1.0462, 6.3678)
  line L652 (1.0462, 6.3678) -> (1.0687, 6.3711)
  line L653 (1.0687, 6.3711) -> (1.0915, 6.3781)
  line L654 (1.0915, 6.3781) -> (1.1144, 6.3889)
  line L655 (1.1144, 6.3889) -> (1.1373, 6.4034)
  line L656 (1.1373, 6.4034) -> (1.1823, 6.4438)
  line L657 (1.1823, 6.4438) -> (1.2253, 6.4992)
  line L658 (1.2253, 6.4992) -> (1.2653, 6.5695)
  line L659 (1.2653, 6.5695) -> (1.301, 6.6545)
  line L660 (1.301, 6.6545) -> (1.3312, 6.754)
  line L661 (1.3312, 6.754) -> (1.3548, 6.8675)
  line L662 (1.3548, 6.8675) -> (1.3638, 6.9241)
  line L663 (1.3638, 6.9241) -> (1.396, 7.0208)
  line L664 (1.396, 7.0208) -> (1.4486, 7.1395)
  line L665 (1.4486, 7.1395) -> (1.4866, 7.2131)
  line L666 (1.4866, 7.2131) -> (1.5342, 7.2963)
  line L667 (1.5342, 7.2963) -> (1.5917, 7.3878)
  line L668 (1.5917, 7.3878) -> (1.6598, 7.4867)
  line L669 (1.6598, 7.4867) -> (1.7411, 7.5949)
  line L670 (1.7411, 7.5949) -> (1.8324, 7.7062)
  line L671 (1.8324, 7.7062) -> (1.9374, 7.8238)
  line L672 (1.9374, 7.8238) -> (2.0556, 7.9456)
  line L673 (2.0556, 7.9456) -> (2.1882, 8.0711)
  line L674 (2.1882, 8.0711) -> (2.3119, 8.1796)
  arc A12 (2.9362, 7.9768) -> (2.3119, 8.1796) centre (0, 0) ccw
  line L675 (2.9362, 7.9768) -> (2.9727, 7.8166)
  line L676 (2.9727, 7.8166) -> (3.0061, 7.6371)
  line L677 (3.0061, 7.6371) -> (3.0302, 7.4691)
  line L678 (3.0302, 7.4691) -> (3.046, 7.3122)
  line L679 (3.046, 7.3122) -> (3.0545, 7.1685)
  line L680 (3.0545, 7.1685) -> (3.0568, 7.0332)
  line L681 (3.0568, 7.0332) -> (3.0537, 6.9131)
  line L682 (3.0537, 6.9131) -> (3.0465, 6.8053)
  line L683 (3.0465, 6.8053) -> (3.0361, 6.71)
  line L684 (3.0361, 6.71) -> (3.0237, 6.6281)
  line L685 (3.0237, 6.6281) -> (2.9964, 6.5012)
  line L686 (2.9964, 6.5012) -> (2.9656, 6.4041)
  line L687 (2.9656, 6.4041) -> (2.9396, 6.353)
  line L688 (2.9396, 6.353) -> (2.892, 6.2472)
  line L689 (2.892, 6.2472) -> (2.858, 6.149)
  line L690 (2.858, 6.149) -> (2.8369, 6.0593)
  line L691 (2.8369, 6.0593) -> (2.8279, 5.9789)
  line L692 (2.8279, 5.9789) -> (2.8302, 5.9088)
  line L693 (2.8302, 5.9088) -> (2.8429, 5.8497)
  line L694 (2.8429, 5.8497) -> (2.8528, 5.8244)
  line L695 (2.8528, 5.8244) -> (2.865, 5.8022)
  line L696 (2.865, 5.8022) -> (2.8793, 5.7832)
  line L697 (2.8793, 5.7832) -> (2.8956, 5.7672)
  line L698 (2.8956, 5.7672) -> (2.9186, 5.7519)
  line L699 (2.9186, 5.7519) -> (3.1517, 5.6276)
  line L700 (3.1517, 5.6276) -> (3.2248, 5.586)
  line L701 (3.2248, 5.586) -> (3.2973, 5.5435)
  line L702 (3.2973, 5.5435) -> (3.5215, 5.4039)
  line L703 (3.5215, 5.4039) -> (3.5463, 5.3916)
  line L704 (3.5463, 5.3916) -> (3.5682, 5.3855)
  line L705 (3.5682, 5.3855) -> (3.5919, 5.3826)
  line L706 (3.5919, 5.3826) -> (3.6172, 5.3832)
  line L707 (3.6172, 5.3832) -> (3.644, 5.3872)
  line L708 (3.644, 5.3872) -> (3.7016, 5.4058)
  line L709 (3.7016, 5.4058) -> (3.7634, 5.4389)
  line L710 (3.7634, 5.4389) -> (3.8285, 5.4869)
  line L711 (3.8285, 5.4869) -> (3.8957, 5.55)
  line L712 (3.8957, 5.55) -> (3.9637, 5.6286)
  line L713 (3.9637, 5.6286) -> (4.0315, 5.7227)
  line L714 (4.0315, 5.7227) -> (4.0627, 5.7708)
  line L715 (4.0627, 5.7708) -> (4.1314, 5.846)
  line L716 (4.1314, 5.846) -> (4.2277, 5.9331)
  line L717 (4.2277, 5.9331) -> (4.2924, 5.9848)
  line L718 (4.2924, 5.9848) -> (4.3697, 6.0414)
  line L719 (4.3697, 6.0414) -> (4.4594, 6.1016)
  line L720 (4.4594, 6.1016) -> (4.5619, 6.1643)
  line L721 (4.5619, 6.1643) -> (4.6803, 6.23)
  line L722 (4.6803, 6.23) -> (4.8089, 6.2946)
  line L723 (4.8089, 6.2946) -> (4.9527, 6.3593)
  line L724 (4.9527, 6.3593) -> (5.1102, 6.4225)
  line L725 (5.1102, 6.4225) -> (5.2824, 6.4833)
  line L726 (5.2824, 6.4833) -> (5.4393, 6.5318)
  arc A13 (5.9265, 6.0931) -> (5.4393, 6.5318) centre (0, 0) ccw
  line L727 (5.9265, 6.0931) -> (5.8947, 5.932)
  line L728 (5.8947, 5.932) -> (5.8523, 5.7544)
  line L729 (5.8523, 5.7544) -> (5.8059, 5.5911)
  line L730 (5.8059, 5.5911) -> (5.7566, 5.4414)
  line L731 (5.7566, 5.4414) -> (5.7059, 5.3066)
  line L732 (5.7059, 5.3066) -> (5.6529, 5.1821)
  line L733 (5.6529, 5.1821) -> (5.6012, 5.0736)
  line L734 (5.6012, 5.0736) -> (5.5508, 4.9781)
  line L735 (5.5508, 4.9781) -> (5.5025, 4.8953)
  line L736 (5.5025, 4.8953) -> (5.4579, 4.8255)
  line L737 (5.4579, 4.8255) -> (5.3814, 4.7206)
  line L738 (5.3814, 4.7206) -> (5.3137, 4.6444)
  line L739 (5.3137, 4.6444) -> (5.2692, 4.6084)
  line L740 (5.2692, 4.6084) -> (5.1827, 4.5311)
  line L741 (5.1827, 4.5311) -> (5.1117, 4.4552)
  line L742 (5.1117, 4.4552) -> (5.0559, 4.3818)
  line L743 (5.0559, 4.3818) -> (5.015, 4.3121)
  line L744 (5.015, 4.3121) -> (4.9885, 4.2471)
  line L745 (4.9885, 4.2471) -> (4.976, 4.1879)
  line L746 (4.976, 4.1879) -> (4.9749, 4.1608)
  line L747 (4.9749, 4.1608) -> (4.977, 4.1356)
  line L748 (4.977, 4.1356) -> (4.9823, 4.1123)
  line L749 (4.9823, 4.1123) -> (4.9907, 4.0912)
  line L750 (4.9907, 4.0912) -> (5.0054, 4.0678)
  line L751 (5.0054, 4.0678) -> (5.1677, 3.8594)
  line L752 (5.1677, 3.8594) -> (5.2176, 3.7917)
  line L753 (5.2176, 3.7917) -> (5.2666, 3.7234)
  line L754 (5.2666, 3.7234) -> (5.4145, 3.5045)
  line L755 (5.4145, 3.5045) -> (5.4321, 3.4833)
  line L756 (5.4321, 3.4833) -> (5.4497, 3.4687)
  line L757 (5.4497, 3.4687) -> (5.4702, 3.4565)
  line L758 (5.4702, 3.4565) -> (5.4935, 3.4467)
  line L759 (5.4935, 3.4467) -> (5.5196, 3.4394)
  line L760 (5.5196, 3.4394) -> (5.5797, 3.433)
  line L761 (5.5797, 3.433) -> (5.6497, 3.4381)
  line L762 (5.6497, 3.4381) -> (5.7287, 3.4554)
  line L763 (5.7287, 3.4554) -> (5.8158, 3.4858)
  line L764 (5.8158, 3.4858) -> (5.9099, 3.5298)
  line L765 (5.9099, 3.5298) -> (6.0101, 3.5883)
  line L766 (6.0101, 3.5883) -> (6.0581, 3.6195)
  line L767 (6.0581, 3.6195) -> (6.1515, 3.6603)
  line L768 (6.1515, 3.6603) -> (6.2749, 3.7006)
  line L769 (6.2749, 3.7006) -> (6.355, 3.7216)
  line L770 (6.355, 3.7216) -> (6.4487, 3.7419)
  line L771 (6.4487, 3.7419) -> (6.5551, 3.7604)
  line L772 (6.5551, 3.7604) -> (6.6742, 3.776)
  line L773 (6.6742, 3.776) -> (6.8091, 3.7879)
  line L774 (6.8091, 3.7879) -> (6.9529, 3.7945)
  line L775 (6.9529, 3.7945) -> (7.1105, 3.7952)
  line L776 (7.1105, 3.7952) -> (7.2801, 3.7888)
  line L777 (7.2801, 3.7888) -> (7.4621, 3.7743)
  line L778 (7.4621, 3.7743) -> (7.6256, 3.755)
  arc A14 (7.8928, 3.155) -> (7.6256, 3.755) centre (0, 0) ccw
  line L779 (7.8928, 3.155) -> (7.7981, 3.0207)
  line L780 (7.7981, 3.0207) -> (7.6871, 2.8757)
  line L781 (7.6871, 2.8757) -> (7.5784, 2.7454)
  line L782 (7.5784, 2.7454) -> (7.4724, 2.6287)
  line L783 (7.4724, 2.6287) -> (7.3713, 2.5262)
  line L784 (7.3713, 2.5262) -> (7.2722, 2.434)
  line L785 (7.2722, 2.434) -> (7.181, 2.3559)
  line L786 (7.181, 2.3559) -> (7.096, 2.2892)
  line L787 (7.096, 2.2892) -> (7.0182, 2.2331)
  line L788 (7.0182, 2.2331) -> (6.9491, 2.1876)
  line L789 (6.9491, 2.1876) -> (6.8365, 2.1229)
  line L790 (6.8365, 2.1229) -> (6.7437, 2.0808)
  line L791 (6.7437, 2.0808) -> (6.6884, 2.066)
  line L792 (6.6884, 2.066) -> (6.5779, 2.0306)
  line L793 (6.5779, 2.0306) -> (6.4822, 1.9901)
  line L794 (6.4822, 1.9901) -> (6.4013, 1.9458)
  line L795 (6.4013, 1.9458) -> (6.3356, 1.8987)
  line L796 (6.3356, 1.8987) -> (6.285, 1.8501)
  line L797 (6.285, 1.8501) -> (6.2496, 1.8011)
  line L798 (6.2496, 1.8011) -> (6.2375, 1.7768)
  line L799 (6.2375, 1.7768) -> (6.2291, 1.7529)
  line L800 (6.2291, 1.7529) -> (6.2245, 1.7295)
  line L801 (6.2245, 1.7295) -> (6.2236, 1.7067)
  line L802 (6.2236, 1.7067) -> (6.2276, 1.6794)
  line L803 (6.2276, 1.6794) -> (6.2912, 1.423)
  line L804 (6.2912, 1.423) -> (6.3092, 1.3409)
  line L805 (6.3092, 1.3409) -> (6.3262, 1.2585)
  line L806 (6.3262, 1.2585) -> (6.3724, 0.9985)
  line L807 (6.3724, 0.9985) -> (6.3799, 0.9719)
  line L808 (6.3799, 0.9719) -> (6.39, 0.9515)
  line L809 (6.39, 0.9515) -> (6.4037, 0.932)
  line L810 (6.4037, 0.932) -> (6.421, 0.9135)
  line L811 (6.421, 0.9135) -> (6.4419, 0.8963)
  line L812 (6.4419, 0.8963) -> (6.4943, 0.8659)
  line L813 (6.4943, 0.8659) -> (6.5603, 0.8421)
  line L814 (6.5603, 0.8421) -> (6.6395, 0.8258)
  line L815 (6.6395, 0.8258) -> (6.7313, 0.8182)
  line L816 (6.7313, 0.8182) -> (6.8353, 0.8202)
  line L817 (6.8353, 0.8202) -> (6.9506, 0.8328)
  line L818 (6.9506, 0.8328) -> (7.0072, 0.8418)
  line L819 (7.0072, 0.8418) -> (7.1091, 0.8411)
  line L820 (7.1091, 0.8411) -> (7.2382, 0.8277)
  line L821 (7.2382, 0.8277) -> (7.3199, 0.8143)
  line L822 (7.3199, 0.8143) -> (7.4138, 0.7947)
  line L823 (7.4138, 0.7947) -> (7.5185, 0.7683)
  line L824 (7.5185, 0.7683) -> (7.6336, 0.7341)
  line L825 (7.6336, 0.7341) -> (7.7617, 0.6901)
  line L826 (7.7617, 0.6901) -> (7.8957, 0.6377)
  line L827 (7.8957, 0.6377) -> (8.04, 0.5742)
  line L828 (8.04, 0.5742) -> (8.1924, 0.4994)
  line L829 (8.1924, 0.4994) -> (8.3528, 0.4121)
  line L830 (8.3528, 0.4121) -> (8.4937, 0.328)
  arc A15 (8.4937, -0.328) -> (8.4937, 0.328) centre (0, 0) ccw
  line L831 (8.4937, -0.328) -> (8.3525, -0.4122)
  line L832 (8.3525, -0.4122) -> (8.1921, -0.4995)
  line L833 (8.1921, -0.4995) -> (8.0398, -0.5743)
  line L834 (8.0398, -0.5743) -> (7.8955, -0.6378)
  line L835 (7.8955, -0.6378) -> (7.7614, -0.6903)
  line L836 (7.7614, -0.6903) -> (7.6334, -0.7343)
  line L837 (7.6334, -0.7343) -> (7.5183, -0.7685)
  line L838 (7.5183, -0.7685) -> (7.4135, -0.7949)
  line L839 (7.4135, -0.7949) -> (7.3197, -0.8145)
  line L840 (7.3197, -0.8145) -> (7.238, -0.828)
  line L841 (7.238, -0.828) -> (7.1089, -0.8413)
  line L842 (7.1089, -0.8413) -> (7.007, -0.842)
  line L843 (7.007, -0.842) -> (6.9504, -0.8331)
  line L844 (6.9504, -0.8331) -> (6.835, -0.8204)
  line L845 (6.835, -0.8204) -> (6.7311, -0.8184)
  line L846 (6.7311, -0.8184) -> (6.6393, -0.8261)
  line L847 (6.6393, -0.8261) -> (6.5601, -0.8424)
  line L848 (6.5601, -0.8424) -> (6.4941, -0.8662)
  line L849 (6.4941, -0.8662) -> (6.4418, -0.8965)
  line L850 (6.4418, -0.8965) -> (6.4209, -0.9138)
  line L851 (6.4209, -0.9138) -> (6.4035, -0.9322)
  line L852 (6.4035, -0.9322) -> (6.3898, -0.9517)
  line L853 (6.3898, -0.9517) -> (6.3797, -0.9722)
  line L854 (6.3797, -0.9722) -> (6.3722, -0.9988)
  line L855 (6.3722, -0.9988) -> (6.326, -1.2588)
  line L856 (6.326, -1.2588) -> (6.309, -1.3412)
  line L857 (6.309, -1.3412) -> (6.291, -1.4233)
  line L858 (6.291, -1.4233) -> (6.2274, -1.6797)
  line L859 (6.2274, -1.6797) -> (6.2234, -1.707)
  line L860 (6.2234, -1.707) -> (6.2243, -1.7298)
  line L861 (6.2243, -1.7298) -> (6.2289, -1.7532)
  line L862 (6.2289, -1.7532) -> (6.2373, -1.7771)
  line L863 (6.2373, -1.7771) -> (6.2493, -1.8014)
  line L864 (6.2493, -1.8014) -> (6.2848, -1.8503)
  line L865 (6.2848, -1.8503) -> (6.3354, -1.899)
  line L866 (6.3354, -1.899) -> (6.4012, -1.946)
  line L867 (6.4012, -1.946) -> (6.482, -1.9904)
  line L868 (6.482, -1.9904) -> (6.5777, -2.0308)
  line L869 (6.5777, -2.0308) -> (6.6882, -2.0662)
  line L870 (6.6882, -2.0662) -> (6.7436, -2.081)
  line L871 (6.7436, -2.081) -> (6.8364, -2.1231)
  line L872 (6.8364, -2.1231) -> (6.9489, -2.1878)
  line L873 (6.9489, -2.1878) -> (7.0181, -2.2333)
  line L874 (7.0181, -2.2333) -> (7.0959, -2.2894)
  line L875 (7.0959, -2.2894) -> (7.1808, -2.3561)
  line L876 (7.1808, -2.3561) -> (7.2721, -2.4341)
  line L877 (7.2721, -2.4341) -> (7.3712, -2.5264)
  line L878 (7.3712, -2.5264) -> (7.4724, -2.6288)
  line L879 (7.4724, -2.6288) -> (7.5784, -2.7455)
  line L880 (7.5784, -2.7455) -> (7.6871, -2.8758)
  line L881 (7.6871, -2.8758) -> (7.7981, -3.0208)
  line L882 (7.7981, -3.0208) -> (7.8928, -3.155)
  arc A16 (7.626, -3.7543) -> (7.8928, -3.155) centre (0, 0) ccw
  line L883 (7.626, -3.7543) -> (7.4628, -3.7736)
  line L884 (7.4628, -3.7736) -> (7.2808, -3.7881)
  line L885 (7.2808, -3.7881) -> (7.1112, -3.7945)
  line L886 (7.1112, -3.7945) -> (6.9535, -3.7939)
  line L887 (6.9535, -3.7939) -> (6.8097, -3.7873)
  line L888 (6.8097, -3.7873) -> (6.6748, -3.7754)
  line L889 (6.6748, -3.7754) -> (6.5557, -3.7598)
  line L890 (6.5557, -3.7598) -> (6.4493, -3.7414)
  line L891 (6.4493, -3.7414) -> (6.3556, -3.721)
  line L892 (6.3556, -3.721) -> (6.2755, -3.7001)
  line L893 (6.2755, -3.7001) -> (6.1521, -3.6598)
  line L894 (6.1521, -3.6598) -> (6.0587, -3.619)
  line L895 (6.0587, -3.619) -> (6.0106, -3.5878)
  line L896 (6.0106, -3.5878) -> (5.9104, -3.5294)
  line L897 (5.9104, -3.5294) -> (5.8163, -3.4853)
  line L898 (5.8163, -3.4853) -> (5.7293, -3.455)
  line L899 (5.7293, -3.455) -> (5.6503, -3.4376)
  line L900 (5.6503, -3.4376) -> (5.5803, -3.4326)
  line L901 (5.5803, -3.4326) -> (5.5202, -3.439)
  line L902 (5.5202, -3.439) -> (5.4941, -3.4462)
  line L903 (5.4941, -3.4462) -> (5.4707, -3.456)
  line L904 (5.4707, -3.456) -> (5.4502, -3.4683)
  line L905 (5.4502, -3.4683) -> (5.4327, -3.4828)
  line L906 (5.4327, -3.4828) -> (5.4151, -3.5041)
  line L907 (5.4151, -3.5041) -> (5.2671, -3.7229)
  line L908 (5.2671, -3.7229) -> (5.2181, -3.7912)
  line L909 (5.2181, -3.7912) -> (5.1682, -3.8589)
  line L910 (5.1682, -3.8589) -> (5.0059, -4.0673)
  line L911 (5.0059, -4.0673) -> (4.9911, -4.0907)
  line L912 (4.9911, -4.0907) -> (4.9827, -4.1119)
  line L913 (4.9827, -4.1119) -> (4.9774, -4.1351)
  line L914 (4.9774, -4.1351) -> (4.9753, -4.1603)
  line L915 (4.9753, -4.1603) -> (4.9765, -4.1874)
  line L916 (4.9765, -4.1874) -> (4.989, -4.2466)
  line L917 (4.989, -4.2466) -> (5.0154, -4.3116)
  line L918 (5.0154, -4.3116) -> (5.0563, -4.3813)
  line L919 (5.0563, -4.3813) -> (5.1121, -4.4547)
  line L920 (5.1121, -4.4547) -> (5.1831, -4.5306)
  line L921 (5.1831, -4.5306) -> (5.2697, -4.6079)
  line L922 (5.2697, -4.6079) -> (5.3142, -4.6439)
  line L923 (5.3142, -4.6439) -> (5.3819, -4.7201)
  line L924 (5.3819, -4.7201) -> (5.4584, -4.825)
  line L925 (5.4584, -4.825) -> (5.503, -4.8947)
  line L926 (5.503, -4.8947) -> (5.5513, -4.9776)
  line L927 (5.5513, -4.9776) -> (5.6018, -5.0731)
  line L928 (5.6018, -5.0731) -> (5.6534, -5.1815)
  line L929 (5.6534, -5.1815) -> (5.7064, -5.3061)
  line L930 (5.7064, -5.3061) -> (5.7571, -5.4408)
  line L931 (5.7571, -5.4408) -> (5.8065, -5.5905)
  line L932 (5.8065, -5.5905) -> (5.8528, -5.7538)
  line L933 (5.8528, -5.7538) -> (5.8953, -5.9314)
  line L934 (5.8953, -5.9314) -> (5.9271, -6.0925)
  arc A17 (5.4396, -6.5315) -> (5.9271, -6.0925) centre (0, 0) ccw
  line L935 (5.4396, -6.5315) -> (5.2825, -6.4827)
  line L936 (5.2825, -6.4827) -> (5.1103, -6.422)
  line L937 (5.1103, -6.422) -> (4.9528, -6.3588)
  line L938 (4.9528, -6.3588) -> (4.809, -6.2941)
  line L939 (4.809, -6.2941) -> (4.6803, -6.2296)
  line L940 (4.6803, -6.2296) -> (4.562, -6.1639)
  line L941 (4.562, -6.1639) -> (4.4595, -6.1012)
  line L942 (4.4595, -6.1012) -> (4.3698, -6.041)
  line L943 (4.3698, -6.041) -> (4.2925, -5.9843)
  line L944 (4.2925, -5.9843) -> (4.2278, -5.9326)
  line L945 (4.2278, -5.9326) -> (4.1315, -5.8456)
  line L946 (4.1315, -5.8456) -> (4.0628, -5.7704)
  line L947 (4.0628, -5.7704) -> (4.0316, -5.7223)
  line L948 (4.0316, -5.7223) -> (3.9638, -5.6282)
  line L949 (3.9638, -5.6282) -> (3.8957, -5.5496)
  line L950 (3.8957, -5.5496) -> (3.8286, -5.4865)
  line L951 (3.8286, -5.4865) -> (3.7635, -5.4385)
  line L952 (3.7635, -5.4385) -> (3.7016, -5.4054)
  line L953 (3.7016, -5.4054) -> (3.644, -5.3869)
  line L954 (3.644, -5.3869) -> (3.6172, -5.3829)
  line L955 (3.6172, -5.3829) -> (3.5919, -5.3823)
  line L956 (3.5919, -5.3823) -> (3.5682, -5.3852)